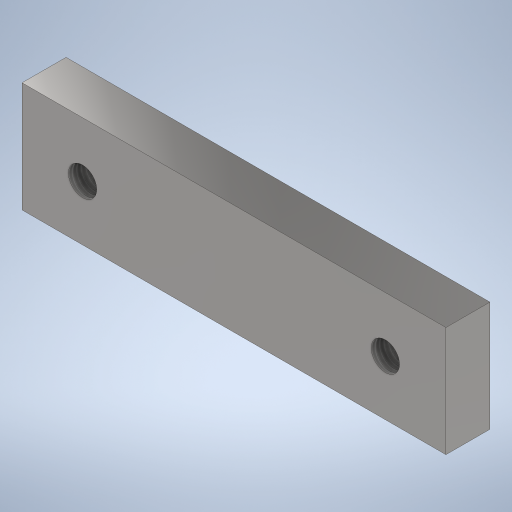
# Autodesk Inventor part: Spann backe
Saved by Autodesk Inventor 2023.2 (Build 272271000, 271)
## iProperties
Created: 2023-02-02
Part Number: Spann backe
Material: Steel, Mild
Document SubType Name: Modeling
Designer: Aditya
Density: 7.85 g/cm^3
Appearance: Semi-Polished
Author: Aditya
Autodesk Inventor part; units mm, degrees
ref_plane "YZ Plane" through (0, 0, 0) normal (1, 0, 0) x (0, 1, 0)
ref_plane "XZ Plane" through (0, 0, 0) normal (0, 1, 0) x (-1, 0, 0)
ref_plane "XY Plane" through (0, 0, 0) normal (0, 0, 1) x (1, 0, 0)
sketch "Sketch1" plane through (0, 0, 0) normal (0, 0, 1) x (1, 0, 0)
  line L0 (-38.5, -10) -> (38.5, -10)
  line L1 (38.5, -10) -> (38.5, 10)
  line L2 (38.5, 10) -> (-38.5, 10)
  line L3 (-38.5, 10) -> (-38.5, -10)
  line L4 (-38.5, -10) -> (38.5, 10) construction
  line L5 (38.5, -10) -> (-38.5, 10) construction
  point P0 (0, 0)
  dimension "d0" = 77
  dimension "d1" = 20
  constraints: 12 end point, 2 midpoint, 2 parallel, 1 horizontal, 1 perpendicular
  measures "d0" distance of L2.end L1.end
  measures "d1" distance of L1.end L0.end
extrude "Extrusion1" add sketch "Sketch1" along normal blind 8
sketch "Sketch2" plane through (0, 0, 8) normal (0, 0, 1) x (1, 0, 0)
  line L0 (-38.5, -10) -> (38.5, -10) projected
  line L1 (38.5, -10) -> (38.5, 10) projected
  line L2 (-38.5, 10) -> (-38.5, -10) projected
  point P0 (0, 0)
  point P1 (-27.5, 0)
  point P2 (27.5, 0)
  point P3 (-38.5, 0)
  dimension "d4" = 10
  dimension "d5" = 10
  dimension "d6" = 11
  dimension "d14" = 11
  constraints: 1 midpoint
  measures "d4" distance from line of L0 point (-27.5, 0)
  measures "d5" distance from line of L0 point (27.5, 0)
  measures "d6" distance from line of L1 point (27.5, 0)
  measures "d14" distance of point (-38.5, 0) point (-27.5, 0)
hole "Hole1" at (-27.5, 0, 8) at (27.5, 0, 8) direction (0, 0, -1) diameter 5.134 depth 6 thread size "M6x0.8" class "6H" standard "ISO Metric profile"
body "Solid1"
